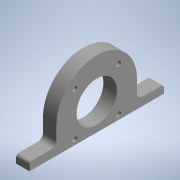
# Autodesk Inventor part: Soporte_Gearbox
Saved by Autodesk Inventor 2022.1 (Build 261234000, 234)
## iProperties
Part Number: Soporte_Gearbox
Material: Genérico
Document SubType Name: Modelado
Designer: seb_0
Appearance: Por defecto
Author: seb_0
Autodesk Inventor part; units mm, degrees
ref_plane "Plano YZ" through (0, 0, 0) normal (1, 0, 0) x (0, 1, 0)
ref_plane "Plano XZ" through (0, 0, 0) normal (0, 1, 0) x (-1, 0, 0)
ref_plane "Plano XY" through (0, 0, 0) normal (0, 0, 1) x (1, 0, 0)
sketch "Boceto1" plane through (0, 0, 0) normal (1, 0, 0) x (0, 1, 0)
  circle A0 centre (0, 0) radius 37.5
  arc A1 (-49.5, -29.2575) -> (-49.5, 29.2575) centre (0, 0) ccw
  line L0 (0, 0) -> (-49.5, 0)
  line L1 (-49.5, 125) -> (-49.5, -125)
  circle A2 centre (40.6586, -40.6586) radius 4.5
  circle A3 centre (40.6586, 40.6586) radius 4.5
  circle A4 centre (-40.6586, 40.6586) radius 4.5
  circle A5 centre (-40.6586, -40.6586) radius 4.5
  line L2 (-40.6586, 40.6586) -> (0, 0)
  line L3 (0, 0) -> (40.6586, -40.6586)
  line L4 (-40.6586, -40.6586) -> (0, 0)
  line L5 (0, 0) -> (40.6586, 40.6586)
  arc A6 (-49.5, -56.3449) -> (-49.5, 56.3449) centre (0, 0) ccw
  line L6 (-49.5, 125) -> (-39.5, 125)
  line L7 (0, 75) -> (-24.5, 75)
  line L8 (-34.5, 85) -> (-34.5, 120)
  line L9 (-49.5, -125) -> (-39.5, -125)
  line L10 (0, -75) -> (-24.5, -75)
  line L11 (-34.5, -85) -> (-34.5, -120)
  arc A7 (-34.5, 85) -> (-24.5, 75) centre (-24.5, 85) ccw
  arc A8 (-24.5, -75) -> (-34.5, -85) centre (-24.5, -85) ccw
  arc A9 (-34.5, 120) -> (-39.5, 125) centre (-39.5, 120) ccw
  arc A10 (-39.5, -125) -> (-34.5, -120) centre (-39.5, -120) ccw
  point P0 (-34.5, 125)
  point P1 (-34.5, -125)
  dimension "d0" = 75
  dimension "d1" = 115
  dimension "d4" = 49.5
  dimension "d5" = 250
  dimension "d11" = 9
  dimension "d12" = 9
  dimension "d13" = 9
  dimension "d14" = 9
  dimension "d15" = 90
  dimension "d16" = 90
  dimension "d17" = 90
  dimension "d19" = 150
  dimension "d20" = 15
  dimension "d21" = 10
  dimension "d22" = 5
  dimension "d23" = 5
  dimension "d24" = 45
  constraints: 24 end point, 18 point on circle, 11 centre point, 10 tangent, 9 point on line, 4 horizontal, 3 coincident, 3 perpendicular, 1 equal radius, 1 midpoint, 1 vertical
  measures "d0" diameter of A0
  measures "d1" diameter of A1
  measures "d4" distance of L0.end L0.start
  measures "d5" distance of L1.start L1.end
  measures "d11" diameter of A2
  measures "d12" diameter of A3
  measures "d13" diameter of A4
  measures "d14" diameter of A5
  measures "d15" angle of L3 L5
  measures "d16" angle of L4 L3
  measures "d17" angle of L2 L4
  measures "d19" diameter of A6
  measures "d20" distance of L1.start point (-34.5, 125)
  measures "d21" radius of A7
  measures "d22" radius of A9
  measures "d23" radius of A10
  measures "d24" angle of L1 L5
extrude "Extrusión1" add sketch "Boceto1" along normal blind 25 contours A0 L5 A3 A1 A2 L3 | A0 L2 A4 A1 A3 L5 | L3 A2 A1 A5 L4 A0 | A0 L0 L1 A1 A4 L2 | L4 A5 A1 L1 L0 A0 | A1 A4 L1 A6 A5 A2 A3 | L1 L6 A9 L8 A7 L7 A6 | A6 L10 A8 L11 A10 L9 L1
